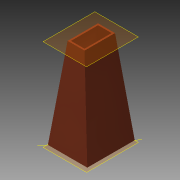
# Autodesk Inventor part: NewHorn
Saved by Autodesk Inventor 2015 (Build 190159000, 159)
## iProperties
Created: 2014-03-24
Part Number: NewHorn
Material: Copper
Document SubType Name: Modeling
Designer: jad211
Density: 8.94 g/cm^3
Appearance: Copper - Satin
Author: jad211
Autodesk Inventor part; units mm, degrees
ref_plane "YZ Plane" through (0, 0, 0) normal (1, 0, 0) x (0, 1, 0)
ref_plane "XZ Plane" through (0, 0, 0) normal (0, 1, 0) x (-1, 0, 0)
ref_plane "XY Plane" through (0, 0, 0) normal (0, 0, 1) x (1, 0, 0)
sketch "Sketch1" plane through (0, 0, 0) normal (0, 0, 1) x (1, 0, 0)
  line L0 (-11.5, -13.85) -> (11.5, -13.85)
  line L1 (11.5, -13.85) -> (11.5, 13.85)
  line L2 (11.5, 13.85) -> (-11.5, 13.85)
  line L3 (-11.5, 13.85) -> (-11.5, -13.85)
  line L4 (-11.5, -13.85) -> (11.5, 13.85) construction
  line L5 (11.5, -13.85) -> (-11.5, 13.85) construction
  point P0 (0, 0)
  dimension "d0" = 23
  dimension "d1" = 27.7
  constraints: 12 end point, 2 midpoint, 2 parallel, 1 horizontal, 1 perpendicular
  measures "d0" distance of L2.end L1.end
  measures "d1" distance of L1.end L0.end
ref_plane "Work Plane2" through (11.5, -13.85, 53.4) normal (0, 0, 1) x (0, 1, 0)
ref_plane "Work Plane1" through (11.5, -13.85, 0) normal (0, 0, 1) x (0, 1, 0)
sketch "Sketch2" plane through (11.5, -13.85, 53.4) normal (0, 0, 1) x (0, 1, 0)
  line L0 (4.9505, 6.5505) -> (22.7495, 6.5505)
  line L1 (22.7495, 6.5505) -> (22.7495, 16.4495)
  line L2 (22.7495, 16.4495) -> (4.9505, 16.4495)
  line L3 (4.9505, 16.4495) -> (4.9505, 6.5505)
  line L4 (4.9505, 6.5505) -> (22.7495, 16.4495) construction
  line L5 (22.7495, 6.5505) -> (4.9505, 16.4495) construction
  point P0 (13.85, 11.5)
  dimension "d3" = 17.799
  dimension "d4" = 9.899
  constraints: 12 end point, 2 midpoint, 2 parallel, 1 horizontal, 1 perpendicular
  measures "d3" distance of L2.end L1.end
  measures "d4" distance of L1.end L0.end
loft "Loft1" add profiles "Sketch2", "Sketch1"
sketch "Sketch4" plane through (11.5, -13.85, 0) normal (0, 0, -1) x (-1, 0, 0)
  line L0 (1.15, 1.3) -> (21.85, 1.3)
  line L1 (21.85, 1.3) -> (21.85, 26.4)
  line L2 (21.85, 26.4) -> (1.15, 26.4)
  line L3 (1.15, 26.4) -> (1.15, 1.3)
  line L4 (1.15, 1.3) -> (21.85, 26.4) construction
  line L5 (21.85, 1.3) -> (1.15, 26.4) construction
  point P0 (11.5, 13.85)
  dimension "d9" = 20.7
  dimension "d10" = 25.1
  constraints: 12 end point, 2 midpoint, 2 parallel, 1 horizontal, 1 perpendicular
  measures "d9" distance of L2.end L1.end
  measures "d10" distance of L1.end L0.end
sketch "Sketch5" plane through (-4.9495, 8.8995, 53.4) normal (0, 0, 1) x (1, 0, 0)
  line L0 (1, -16.799) -> (8.899, -16.799)
  line L1 (8.899, -16.799) -> (8.899, -1)
  line L2 (8.899, -1) -> (1, -1)
  line L3 (1, -1) -> (1, -16.799)
  line L4 (1, -16.799) -> (8.899, -1) construction
  line L5 (8.899, -16.799) -> (1, -1) construction
  point P0 (4.9495, -8.8995)
  dimension "d11" = 7.899
  dimension "d12" = 15.799
  constraints: 12 end point, 2 midpoint, 2 parallel, 1 horizontal, 1 perpendicular
  measures "d11" distance of L2.end L1.end
  measures "d12" distance of L1.end L0.end
loft "Loft2" cut profiles "Sketch5", "Sketch4"
body "Solid1"
